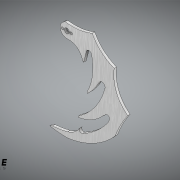
# Autodesk Inventor part: 横回転鎌
Saved by Autodesk Inventor 2020 (Build 240168000, 168)
## iProperties
Created: 2020-02-26
Part Number: 横回転鎌
Material: アルミニウム 7075
Document SubType Name: Modeling
Designer: tanjihayato
Density: 2.81 g/cm^3
Appearance: サテン - ブラシ仕上げ 重厚
Mass: 71.0339 g
Surface Area: 160.013 cm^2
Volume: 25.279 cm^3
Author: tanjihayato
Autodesk Inventor part; units mm, degrees
ref_plane "YZ Plane" through (0, 0, 0) normal (1, 0, 0) x (0, 1, 0)
ref_plane "XZ Plane" through (0, 0, 0) normal (0, 1, 0) x (-1, 0, 0)
ref_plane "XY Plane" through (0, 0, 0) normal (0, 0, 1) x (1, 0, 0)
sketch "スケッチ1" plane through (0, 0, 0) normal (0, 0, 1) x (1, 0, 0)
  circle A0 centre (0, 0) radius 4
  arc A1 (-36.3828, -145.5208) -> (1.7098, -149.9903) centre (0, 0) ccw
  arc A2 (-36.3828, -145.5208) -> (66.3592, -96.2219) centre (-30.943, -25.1476) ccw
  arc A3 (14.4829, -112.8585) -> (61.7505, -49.6452) centre (-38.6267, -23.8672) ccw
  arc A4 (14.4829, -112.8585) -> (58.5345, -90.0081) centre (7.974, -46.4235) ccw
  arc A5 (66.3592, -96.2219) -> (58.5345, -90.0081) centre (62.3217, -93.2727) ccw
  arc A6 (1.2269, -141.2699) -> (20.4921, -126.6173) centre (-7.4844, -109.8252) ccw
  arc A7 (20.4921, -126.6173) -> (25.3099, -131.707) centre (23.6114, -128.4896) ccw
  arc A8 (1.7098, -149.9903) -> (99.9398, -73.8138) centre (-15.6029, -26.2431) ccw
  arc A9 (99.9398, -73.8138) -> (-6.5865, 8.8101) centre (35.2818, -47.1931) ccw
  circle A10 centre (0, 0) radius 11
  circle A11 centre (0, 0) radius 7
  circle A12 centre (-7, 0) radius 2
  circle A13 centre (7, 0) radius 2
  arc A14 (25.6, -35.3039) -> (1.0693, -10.9479) centre (3.2508, -33.2821) ccw
  arc A15 (25.6, -35.3039) -> (31.6019, -13.0505) centre (-166.9688, 28.5691) ccw
  arc A16 (39.8947, -12.9328) -> (31.6019, -13.0505) centre (35.7615, -13.9224) ccw
  arc A17 (29.3196, -75.0304) -> (39.8947, -12.9328) centre (-38.0836, -31.6026) ccw
  arc A18 (29.3196, -75.0304) -> (52.4911, -46.0576) centre (-35.7899, 0.7942) ccw
  arc A19 (61.7505, -49.6452) -> (52.4911, -46.0576) centre (56.9076, -48.4015) ccw
  line L0 (-7, 0) -> (7, 0)
  dimension "d0" = 8
  dimension "d1" = 300
  dimension "d2" = 10
  dimension "d3" = 7
  dimension "d4" = 3
  dimension "d5" = 4
  dimension "d6" = 4
  dimension "d7" = 8.5
  dimension "d8" = 10
  constraints: 36 point on circle, 20 centre point, 12 tangent, 2 coincident, 2 end point, 1 horizontal, 1 horizontal alignment, 1 midpoint
  measures "d0" diameter of A0
  measures "d1" diameter of A1
  measures "d2" diameter of A5
  measures "d3" radial gap between concentric circles of A0 A10
  measures "d4" radial gap between concentric circles of A0 A11
  measures "d5" diameter of A12
  measures "d6" diameter of A13
  measures "d7" diameter of A16
  measures "d8" diameter of A19
extrude "押し出し1" add sketch "スケッチ1" along normal blind 4 contours L0 A13 A11 A12 A0 | A0 L0 A12 A11 A13 | A2 A5 A4 A3 A19 A18 A17 A16 A15 A14 A10 A9 A8 A1 | A6 A7 A2 | A10
sketch "スケッチ2" plane through (0, 0, 4) normal (0, 0, 1) x (1, 0, 0)
  arc A0 (99.9398, -73.8138) -> (-6.5865, 8.8101) centre (35.2818, -47.1931) ccw projected
  arc A1 (-6.5865, 8.8101) -> (1.0693, -10.9479) centre (0, 0) ccw projected
  arc A2 (25.6, -35.3039) -> (1.0693, -10.9479) centre (3.2508, -33.2821) ccw projected
  arc A3 (25.6, -35.3039) -> (31.6019, -13.0505) centre (-166.9688, 28.5691) ccw projected
  arc A4 (39.8947, -12.9328) -> (31.6019, -13.0505) centre (35.7615, -13.9224) ccw projected
  arc A5 (29.3196, -75.0304) -> (39.8947, -12.9328) centre (-38.0836, -31.6026) ccw projected
  arc A6 (29.3196, -75.0304) -> (52.4911, -46.0576) centre (-35.7899, 0.7942) ccw projected
  arc A7 (61.7505, -49.6452) -> (52.4911, -46.0576) centre (56.9076, -48.4015) ccw projected
  arc A8 (14.4829, -112.8585) -> (61.7505, -49.6452) centre (-38.6267, -23.8672) ccw projected
  arc A9 (14.4829, -112.8585) -> (58.5345, -90.0081) centre (7.974, -46.4235) ccw projected
  arc A10 (66.3592, -96.2219) -> (58.5345, -90.0081) centre (62.3217, -93.2727) ccw projected
  arc A11 (25.3099, -131.707) -> (66.3592, -96.2219) centre (-30.943, -25.1476) ccw projected
  arc A12 (20.4921, -126.6173) -> (25.3099, -131.707) centre (23.6114, -128.4896) ccw projected
  arc A13 (1.2269, -141.2699) -> (20.4921, -126.6173) centre (-7.4844, -109.8252) ccw projected
  arc A14 (-36.3828, -145.5208) -> (1.2269, -141.2699) centre (-30.943, -25.1476) ccw projected
  arc A15 (-36.3828, -145.5208) -> (1.7098, -149.9903) centre (0, 0) ccw projected
  arc A16 (1.7098, -149.9903) -> (99.9398, -73.8138) centre (-15.6029, -26.2431) ccw projected
  circle A17 centre (7, 0) radius 2 projected
  circle A18 centre (0, 0) radius 4 projected
  circle A19 centre (-7, 0) radius 2 projected
  circle A20 centre (65.3374, -89.2845) radius 4
  arc A21 (66.3592, -96.2219) -> (58.5345, -90.0081) centre (62.3217, -93.2727) ccw projected
  line L0 (60.732, -88.5321) -> (62.2857, -86.6986)
  line L1 (67.3012, -93.7246) -> (68.7437, -91.3815)
  arc A22 (14.4829, -112.8585) -> (58.5345, -90.0081) centre (7.974, -46.4235) ccw projected
  arc A23 (25.3099, -131.707) -> (66.3592, -96.2219) centre (-30.943, -25.1476) ccw projected
  arc A24 (99.9398, -73.8138) -> (-6.5865, 8.8101) centre (35.2818, -47.1931) ccw projected
  arc A25 (82.9132, 3.9984) -> (100.781, -71.6713) centre (134.0667, -23.8672) ccw
  arc A26 (103.3216, -63.3146) -> (78.1365, -108.8628) centre (240.1923, -168.732) ccw
  arc A27 (-2.9127, 11.3773) -> (49.5081, 21.2681) centre (9, 92.0999) ccw
  line L2 (-23.554, -145.4168) -> (-27.6421, -147.431)
  line L3 (19.0618, -109.9609) -> (18.1257, -112.4002)
  arc A28 (29.3196, -75.0304) -> (39.8947, -12.9328) centre (-38.0836, -31.6026) ccw projected
  line L4 (32.9312, -68.8325) -> (33.161, -71.5549)
  line L5 (25.3099, -29.1624) -> (27.0784, -30.661)
  arc A29 (99.9398, -73.8138) -> (-6.5865, 8.8101) centre (35.2818, -47.1931) ccw projected
  arc A30 (38.5914, 22.6522) -> (98.9338, -18.2494) centre (98.6238, 46.2558) ccw
  point P0 (60.732, -88.5321)
  point P1 (61.4482, -88.3496)
  point P2 (67.2965, -92.7719)
  point P3 (67.3012, -93.7246)
  point P4 (103.3216, -63.3146)
  point P5 (82.9132, 3.9984)
  point P6 (100.781, -71.6713)
  point P7 (-2.9127, 11.3773)
  point P8 (49.5081, 21.2681)
  point P9 (38.5914, 22.6522)
  point P10 (98.9338, -18.2494)
  dimension "d11" = 8
  constraints: 27 point on circle, 12 end point, 5 centre point, 2 tangent, 6 other
  measures "d11" diameter of A20
extrude "押し出し2" cut sketch "スケッチ2" against normal blind 4 contours A16 A26 A25 A0 | A25 A26 A0 | A26 A25 A30 A0 | A30 A25 A0 | A30 A27 A0 A25 | A15 A14 L2 | A30 A0 A27 | A27 A0 A30 | L5 A3 A2 | A10 A20 L1 | A20 A10 | A10 A20 | A10 L0 A20 | L4 A6 A5 | A9 A8 L3
